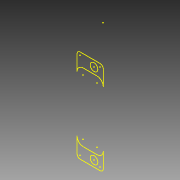
# Autodesk Inventor part: IO-Shield-Topplate01
Saved by Autodesk Inventor 2013 (Build 170138000, 138)
## iProperties
Created: 2015-02-10
Part Number: IO-Shield-Topplate01
Material: Generic
Document SubType Name: Modeling
Designer: spichelh
Density: 1 g/cm^3
Author: spichelh
Autodesk Inventor part; units mm, degrees
ref_plane "YZ Plane" through (0, 0, 0) normal (1, 0, 0) x (0, 1, 0)
ref_plane "XZ Plane" through (0, 0, 0) normal (0, 1, 0) x (-1, 0, 0)
ref_plane "XY Plane" through (0, 0, 0) normal (0, 0, 1) x (1, 0, 0)
sketch "Sketch1" plane through (0, 0, 0) normal (0, 0, 1) x (1, 0, 0)
  arc A0 (-8.5, -36) -> (-6.5, -38) centre (-6.5, -36) ccw construction
  line L0 (-8.5, -40) -> (-8.5, -36) construction
  arc A1 (-8.5, -40) -> (-6.5, -42) centre (-6.5, -40) ccw construction
  line L1 (-2, -42) -> (-6.5, -42) construction
  arc A2 (-2, -42) -> (0, -40) centre (-2, -40) ccw construction
  line L2 (0, -36) -> (0, -40) construction
  arc A3 (-2, -38) -> (0, -36) centre (-2, -36) ccw construction
  line L3 (-2, -38) -> (-6.5, -38) construction
  circle A4 centre (-2, -40) radius 1.25 construction
  circle A5 centre (-2, -13.9) radius 1.25 construction
  arc A6 (-6.5, -15.9) -> (-8.5, -17.9) centre (-6.5, -17.9) ccw construction
  line L4 (-6.5, -15.9) -> (-2, -15.9) construction
  arc A7 (0, -17.9) -> (-2, -15.9) centre (-2, -17.9) ccw construction
  line L5 (0, -13.9) -> (0, -17.9) construction
  arc A8 (0, -13.9) -> (-2, -11.9) centre (-2, -13.9) ccw construction
  line L6 (-6.5, -11.9) -> (-2, -11.9) construction
  arc A9 (-6.5, -11.9) -> (-8.5, -13.9) centre (-6.5, -13.9) ccw construction
  line L7 (-8.5, -17.9) -> (-8.5, -13.9) construction
  line L8 (-6.5, -11.9) -> (-2, -11.9)
  line L9 (0, -13.9) -> (0, -40)
  line L10 (-2, -42) -> (-6.5, -42)
  line L11 (-8.5, -40) -> (-8.5, -13.9)
  arc A10 (-6.5, -11.9) -> (-8.5, -13.9) centre (-6.5, -13.9) ccw
  arc A11 (0, -13.9) -> (-2, -11.9) centre (-2, -13.9) ccw
  arc A12 (-2, -42) -> (0, -40) centre (-2, -40) ccw
  arc A13 (-8.5, -40) -> (-6.5, -42) centre (-6.5, -40) ccw
  circle A14 centre (-2, -13.9) radius 1.25
  circle A15 centre (-2, -40) radius 1.25
  point P0 (0, 0)
  dimension "d0" = 2
  constraints: 8 end point, 8 point on circle, 8 tangent, 6 centre point, 5 equal radius, 2 coincident, 2 parallel, 1 horizontal, 1 perpendicular
  measures "d0" radius of A10
extrude "Extrusion1" add sketch "Sketch1" along normal blind 1
sketch "Sketch2" plane through (0, 0, 0) normal (0, 0, -1) x (-1, 0, 0)
  line L0 (8.5, -13.9) -> (8.5, -40) projected
  line L1 (2, -11.9) -> (6.5, -11.9) projected
  line L2 (0, -40) -> (0, -13.9) projected
  line L3 (6.5, -42) -> (2, -42) projected
  line L4 (2, -15.9) -> (6.5, -15.9)
  line L5 (8.5, -17.9) -> (8.5, -36)
  line L6 (6.5, -38) -> (2, -38)
  line L7 (0, -36) -> (0, -17.9)
  arc A0 (2, -15.9) -> (0, -17.9) centre (2, -17.9) ccw
  arc A1 (8.5, -17.9) -> (6.5, -15.9) centre (6.5, -17.9) ccw
  arc A2 (6.5, -38) -> (8.5, -36) centre (6.5, -36) ccw
  arc A3 (0, -36) -> (2, -38) centre (2, -36) ccw
  point P0 (0, 0)
  point P1 (0, -15.9)
  point P2 (8.5, -38)
  dimension "d3" = 2
  dimension "d4" = 4
  dimension "d5" = 4
  constraints: 8 end point, 8 point on circle, 8 tangent, 6 point on line, 4 centre point, 3 equal radius, 2 parallel, 1 horizontal, 1 perpendicular
  measures "d3" radius of A0
  measures "d4" distance between parallel lines of L3 L6
  measures "d5" distance between parallel lines of L1 L4
extrude "Extrusion2" add sketch "Sketch2" along normal blind 1
chamfer "Chamfer1" distance 0.5 angle 45 18 edges at (-0.5858, -16.4858, -1) (0, -26.95, -1) (-0.5858, -37.4142, -1) (-4.25, -38, -1) (-7.9142, -37.4142, -1) (-8.5, -26.95, -1) (-7.9142, -16.4858, -1) (-4.25, -15.9, -1) (0, -15.9, 0) (-0.5858, -12.4858, 0) (-4.25, -11.9, 0) (-7.9142, -12.4858, 0) (-8.5, -15.9, 0) (-0.5858, -41.4142, 0) (0, -38, 0) (-4.25, -42, 0) (-7.9142, -41.4142, 0) (-8.5, -38, 0)
body "Solid1"
